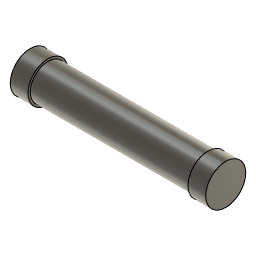
connector v2 (Autodesk Fusion 360 design; units mm, degrees)
Autodesk Fusion 360 part; units mm, degrees
sketch "Sketch1" plane through (0, 0, 0) normal (1, 0, 0) x (0, 1, 0)
  circle A0 centre (0, 0) radius 4.5
  dimension "d1" = 9
  constraint coincident A0.centre origin
  measures "d1" diameter of A0
extrude "Extrude1" add sketch "Sketch1" along normal mid plane 44
sketch "Sketch3" plane through (0, 0, 0) normal (1, 0, 0) x (0, 1, 0)
  circle A0 centre (0, 0) radius 4
  circle A1 centre (0, 0) radius 5
  dimension "d7" = 8
  dimension "d8" = 10
  constraint coincident A0.centre A1.centre
  constraint concentric A0 A1
  measures "d7" diameter of A0
  measures "d8" diameter of A1
extrude "Extrude2" cut sketch "Sketch3" along normal mid plane 36
